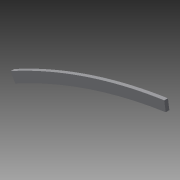
# Autodesk Inventor part: nd-h
Saved by Autodesk Inventor 2015 (Build 190159000, 159)
## iProperties
Created: 2014-07-02
Part Number: nd-h
Material: Generic
Document SubType Name: Modeling
Designer: peter
Density: 1 g/cm^3
Appearance: Default
Author: peter
Autodesk Inventor part; units mm, degrees
ref_plane "YZ Plane" through (0, 0, 0) normal (1, 0, 0) x (0, 1, 0)
ref_plane "XZ Plane" through (0, 0, 0) normal (0, 1, 0) x (-1, 0, 0)
ref_plane "XY Plane" through (0, 0, 0) normal (0, 0, 1) x (1, 0, 0)
sketch "Sketch1" plane through (0, 0, 0) normal (0, 0, 1) x (1, 0, 0)
  line L0 (808.7265, 315.541) -> (816.1873, 265.2919)
  arc A0 (816.1873, 265.2919) -> (24.2674, 0.0436) centre (1166.8448, -2096.4179) ccw
  line L1 (24.2674, 0.0436) -> (-0.0427, 44.6491)
  arc A1 (808.7265, 315.541) -> (-0.0427, 44.6491) centre (1166.8448, -2096.4179) ccw
  point P0 (0, 0)
  constraints: 4 end point, 4 point on circle, 2 centre point
extrude "Extrusion1" add sketch "Sketch1" along normal blind 19.05
body "Solid1"
